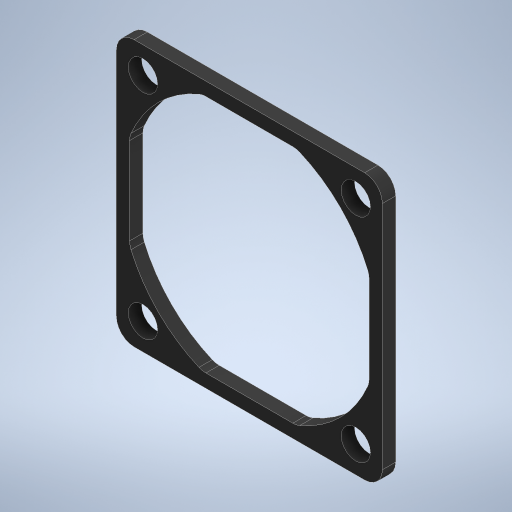
# Autodesk Inventor part: Hotend Cooling Fan Bracket
Saved by Autodesk Inventor 2024 (Build 280153000, 153)
## iProperties
Created: 2025-01-11
Part Number: Hotend Cooling Fan Bracket
Material: Rubber
Document SubType Name: Modeling
Designer: Ishaan
Density: 0.93 g/cm^3
Appearance: Rubber - Black
Author: Ishaan
Autodesk Inventor part; units mm, degrees
ref_plane "YZ Plane" through (0, 0, 0) normal (1, 0, 0) x (0, 1, 0)
ref_plane "XZ Plane" through (0, 0, 0) normal (0, 1, 0) x (-1, 0, 0)
ref_plane "XY Plane" through (0, 0, 0) normal (0, 0, 1) x (1, 0, 0)
sketch "Sketch1" plane through (0, 0, 0) normal (0, 0, 1) x (1, 0, 0)
  line L0 (-15, -15) -> (15, -15)
  line L1 (15, -15) -> (15, 15)
  line L2 (15, 15) -> (-15, 15)
  line L3 (-15, 15) -> (-15, -15)
  line L4 (-15, -15) -> (15, 15) construction
  line L5 (15, -15) -> (-15, 15) construction
  line L6 (-13.5, -13.5) -> (13.5, -13.5)
  line L7 (13.5, -13.5) -> (13.5, 13.5)
  line L8 (13.5, 13.5) -> (-13.5, 13.5)
  line L9 (-13.5, 13.5) -> (-13.5, -13.5)
  line L10 (-13.5, -13.5) -> (13.5, 13.5) construction
  line L11 (13.5, -13.5) -> (-13.5, 13.5) construction
  circle A0 centre (0, 0) radius 14.5
  point P0 (5.2915, -13.5)
  point P1 (-5.2915, -13.5)
  point P2 (-13.5, -5.2915)
  point P3 (-13.5, 5.2915)
  point P4 (-5.2915, 13.5)
  point P5 (5.2915, 13.5)
  point P6 (13.5, 5.2915)
  point P7 (13.5, -5.2915)
  dimension "d0" = 30
  dimension "d1" = 30
  dimension "d2" = 27
  dimension "d3" = 27
  dimension "d4" = 29
  constraints: 24 end point, 4 midpoint, 4 parallel, 2 horizontal, 2 perpendicular, 1 centre point, 1 coincident
  measures "d0" distance of L2.end L1.end
  measures "d1" distance of L1.end L0.end
  measures "d2" distance of L8.end L7.end
  measures "d3" distance of L7.end L6.end
  measures "d4" diameter of A0
extrude "Extrusion1" add sketch "Sketch1" along normal blind 1.5 contours L3 L2 L1 L0 | L9 A0 L6 | L6 A0 | A0 L9 | A0 L7 L6 | L9 L8 A0 | L7 A0 | A0 L8 | A0 L8 L7
fillet "Fillet1" radius 2 12 edges at (15, -15, 0.75) (15, 15, 0.75) (5.2915, 13.5, 0.75) (-13.5, 5.2915, 0.75) (-15, -15, 0.75) (-15, 15, 0.75) (13.5, 5.2915, 0.75) (-5.2915, 13.5, 0.75) (-5.2915, -13.5, 0.75) (-13.5, -5.2915, 0.75) (5.2915, -13.5, 0.75) (13.5, -5.2915, 0.75)
sketch "Sketch2" plane through (0, 0, 1.5) normal (0, 0, 1) x (1, 0, 0)
  line L0 (-12, -12) -> (12, -12) construction
  line L1 (12, -12) -> (12, 12) construction
  line L2 (12, 12) -> (-12, 12) construction
  line L3 (-12, 12) -> (-12, -12) construction
  line L4 (-12, -12) -> (12, 12) construction
  line L5 (12, -12) -> (-12, 12) construction
  point P0 (0, 0)
  dimension "d8" = 24
  dimension "d9" = 24
  constraints: 12 end point, 4 coincident, 2 midpoint, 2 parallel, 1 horizontal, 1 perpendicular
  measures "d8" distance of L2.end L1.end
  measures "d9" distance of L1.end L0.end
hole "Hole1" at (-12, 12, 1.5) at (12, 12, 1.5) at (12, -12, 1.5) at (-12, -12, 1.5) direction (0, 0, -1) diameter 3.3 end through all
body "Solid1"
